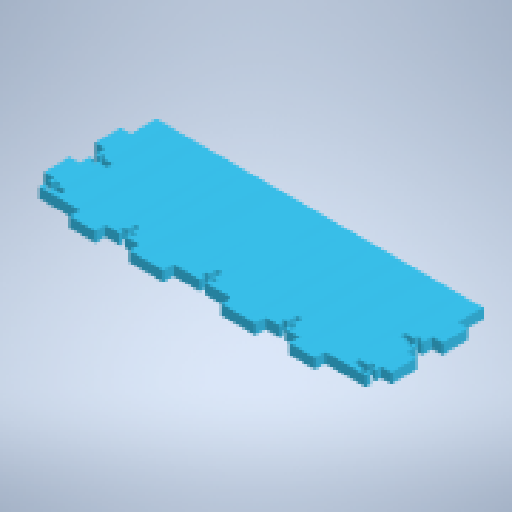
# Autodesk Inventor part: задняя стенка
Saved by Autodesk Inventor 2024.2 (Build 282272000, 272)
## iProperties
Created: 2026-02-22
Part Number: задняя стенка
Material: Типовые
Document SubType Name: Modeling
Designer: Service
Density: 1 g/cm^3
Appearance: Бирюзовый
Author: Service
Autodesk Inventor part; units mm, degrees
ref_plane "YZ Plane" through (0, 0, 0) normal (1, 0, 0) x (0, 1, 0)
ref_plane "XZ Plane" through (0, 0, 0) normal (0, 1, 0) x (-1, 0, 0)
ref_plane "XY Plane" through (0, 0, 0) normal (0, 0, 1) x (1, 0, 0)
sketch "Эскиз1" plane through (0, 0, 0) normal (0, 1, 0) x (-1, 0, 0)
  line L0 (-293.7591, 342.3304) -> (-89.7591, 342.3304)
  line L1 (-89.7591, 342.3304) -> (-89.7591, 402.3304)
  line L2 (-89.7591, 402.3304) -> (-293.7591, 402.3304)
  line L3 (-293.7591, 402.3304) -> (-293.7591, 342.3304)
  line L4 (-293.7591, 387.3304) -> (-287.7591, 387.3304)
  line L5 (-287.7591, 387.3304) -> (-287.7591, 402.3304)
  line L6 (-287.7591, 402.3304) -> (-293.7591, 402.3304)
  line L7 (-293.7591, 402.3304) -> (-293.7591, 387.3304)
  line L8 (-287.7591, 387.3304) -> (-293.7591, 387.3304)
  line L9 (-293.7591, 387.3304) -> (-293.7591, 372.3304)
  line L10 (-293.7591, 372.3304) -> (-287.7591, 372.3304)
  line L11 (-287.7591, 372.3304) -> (-287.7591, 387.3304)
  line L12 (-293.7591, 372.3304) -> (-287.7591, 372.3304)
  line L13 (-287.7591, 372.3304) -> (-287.7591, 357.3304)
  line L14 (-287.7591, 357.3304) -> (-293.7591, 357.3304)
  line L15 (-293.7591, 357.3304) -> (-293.7591, 372.3304)
  line L16 (-287.7591, 357.3304) -> (-293.7591, 357.3304)
  line L17 (-293.7591, 357.3304) -> (-293.7591, 342.3304)
  line L18 (-293.7591, 342.3304) -> (-287.7591, 342.3304)
  line L19 (-287.7591, 342.3304) -> (-287.7591, 357.3304)
  line L20 (-95.7591, 402.3304) -> (-89.7591, 402.3304)
  line L21 (-89.7591, 402.3304) -> (-89.7591, 387.3304)
  line L22 (-89.7591, 387.3304) -> (-95.7591, 387.3304)
  line L23 (-95.7591, 387.3304) -> (-95.7591, 402.3304)
  line L24 (-95.7591, 387.3304) -> (-89.7591, 387.3304)
  line L25 (-89.7591, 387.3304) -> (-89.7591, 372.3304)
  line L26 (-89.7591, 372.3304) -> (-95.7591, 372.3304)
  line L27 (-95.7591, 372.3304) -> (-95.7591, 387.3304)
  line L28 (-95.7591, 372.3304) -> (-89.7591, 372.3304)
  line L29 (-89.7591, 372.3304) -> (-89.7591, 357.3304)
  line L30 (-89.7591, 357.3304) -> (-95.7591, 357.3304)
  line L31 (-95.7591, 357.3304) -> (-95.7591, 372.3304)
  line L32 (-95.7591, 357.3304) -> (-89.7591, 357.3304)
  line L33 (-89.7591, 357.3304) -> (-89.7591, 342.3304)
  line L34 (-89.7591, 342.3304) -> (-95.7591, 342.3304)
  line L35 (-95.7591, 342.3304) -> (-95.7591, 357.3304)
  line L36 (-119.7591, 396.3304) -> (-119.7591, 402.3304)
  line L37 (-89.7591, 390.8181) -> (-89.7591, 394.8304)
  line L38 (-119.7591, 396.3304) -> (-134.7591, 396.3304)
  line L39 (-134.7591, 396.3304) -> (-134.7591, 402.3304)
  line L40 (-134.7591, 402.3304) -> (-119.7591, 402.3304)
  line L41 (-134.7591, 396.3304) -> (-154.7591, 396.3304)
  line L42 (-154.7591, 396.3304) -> (-154.7591, 402.3304)
  line L43 (-154.7591, 402.3304) -> (-134.7591, 402.3304)
  line L44 (-134.7591, 402.3304) -> (-134.7591, 396.3304)
  line L45 (-191.7591, 402.3304) -> (-154.7591, 402.3304)
  line L46 (-154.7591, 402.3304) -> (-154.7591, 396.3304)
  line L47 (-119.7591, 396.3304) -> (-89.7591, 396.3304)
  line L48 (-89.7591, 396.3304) -> (-89.7591, 402.3304)
  line L49 (-89.7591, 402.3304) -> (-119.7591, 402.3304)
  line L50 (-119.7591, 402.3304) -> (-119.7591, 396.3304)
  line L51 (-154.7591, 396.3304) -> (-174.7591, 396.3304)
  line L52 (-174.7591, 396.3304) -> (-174.7591, 402.3304)
  line L53 (-174.7591, 402.3304) -> (-154.7591, 402.3304)
  line L54 (-154.7591, 402.3304) -> (-154.7591, 396.3304)
  line L55 (-293.7591, 394.4817) -> (-263.7591, 394.4817)
  line L56 (-263.7591, 394.4817) -> (-263.7591, 402.3304)
  line L57 (-263.7591, 402.3304) -> (-293.7591, 402.3304)
  line L58 (-293.7591, 402.3304) -> (-293.7591, 394.4817)
  line L59 (-263.7591, 394.4817) -> (-248.7591, 394.4817)
  line L60 (-248.7591, 394.4817) -> (-248.7591, 402.3304)
  line L61 (-248.7591, 402.3304) -> (-263.7591, 402.3304)
  line L62 (-263.7591, 402.3304) -> (-263.7591, 394.4817)
  line L63 (-248.7591, 394.4817) -> (-228.7591, 394.4817)
  line L64 (-228.7591, 394.4817) -> (-228.7591, 402.3304)
  line L65 (-228.7591, 402.3304) -> (-248.7591, 402.3304)
  line L66 (-248.7591, 402.3304) -> (-248.7591, 394.4817)
  line L67 (-228.7591, 394.4817) -> (-208.7591, 394.4817)
  line L68 (-208.7591, 394.4817) -> (-208.7591, 402.3304)
  line L69 (-208.7591, 402.3304) -> (-228.7591, 402.3304)
  line L70 (-228.7591, 402.3304) -> (-228.7591, 394.4817)
  line L71 (-174.7591, 396.3304) -> (-210.3193, 394.4817)
  line L72 (-263.7591, 402.3304) -> (-248.7591, 402.3304)
  line L73 (-248.7591, 402.3304) -> (-248.7591, 417.3304)
  line L74 (-248.7591, 417.3304) -> (-263.7591, 417.3304)
  line L75 (-263.7591, 417.3304) -> (-263.7591, 402.3304)
  line L76 (-228.7591, 402.3304) -> (-208.7591, 402.3304)
  line L77 (-208.7591, 402.3304) -> (-208.7591, 417.3304)
  line L78 (-208.7591, 417.3304) -> (-228.7591, 417.3304)
  line L79 (-228.7591, 417.3304) -> (-228.7591, 402.3304)
  line L80 (-174.7591, 402.3304) -> (-154.7591, 402.3304)
  line L81 (-154.7591, 402.3304) -> (-154.7591, 417.3304)
  line L82 (-154.7591, 417.3304) -> (-174.7591, 417.3304)
  line L83 (-174.7591, 417.3304) -> (-174.7591, 402.3304)
  line L84 (-134.7591, 402.3304) -> (-119.7591, 402.3304)
  line L85 (-119.7591, 402.3304) -> (-119.7591, 417.3304)
  line L86 (-119.7591, 417.3304) -> (-134.7591, 417.3304)
  line L87 (-134.7591, 417.3304) -> (-134.7591, 402.3304)
  line L88 (-95.7591, 402.3304) -> (-95.7591, 411.3304)
  line L89 (-95.7591, 411.3304) -> (-95.7591, 402.3304)
  line L90 (-95.7591, 411.3304) -> (-287.7591, 411.3304)
  line L91 (-287.7591, 411.3304) -> (-287.7591, 402.3304)
  line L92 (-240.2591, 411.3304) -> (-237.2591, 411.3304)
  line L93 (-237.2591, 411.3304) -> (-237.2591, 401.3304)
  line L94 (-237.2591, 401.3304) -> (-240.2591, 401.3304)
  line L95 (-240.2591, 401.3304) -> (-240.2591, 411.3304)
  line L96 (-235.2591, 409.3304) -> (-242.2591, 409.3304)
  line L97 (-242.2591, 409.3304) -> (-242.2591, 406.9304)
  line L98 (-242.2591, 406.9304) -> (-235.2591, 406.9304)
  line L99 (-235.2591, 406.9304) -> (-235.2591, 409.3304)
  line L100 (-190.2591, 411.3304) -> (-190.2591, 401.3304)
  line L101 (-190.2591, 401.3304) -> (-193.2591, 401.3304)
  line L102 (-193.2591, 401.3304) -> (-193.2591, 411.3304)
  line L103 (-188.2591, 408.4317) -> (-195.2591, 408.4317)
  line L104 (-195.2591, 408.4317) -> (-195.2591, 406.0317)
  line L105 (-195.2591, 406.0317) -> (-188.2591, 406.0317)
  line L106 (-188.2591, 406.0317) -> (-188.2591, 408.4317)
  line L107 (-143.2591, 411.3304) -> (-143.2591, 401.3304)
  line L108 (-143.2591, 401.3304) -> (-146.2591, 401.3304)
  line L109 (-146.2591, 401.3304) -> (-146.2591, 404.4797)
  line L110 (-141.2591, 409.3304) -> (-148.2591, 409.3304)
  line L111 (-148.2591, 409.3304) -> (-148.2591, 406.9304)
  line L112 (-148.2591, 406.9304) -> (-141.2591, 406.9304)
  line L113 (-141.2591, 406.9304) -> (-141.2591, 409.3304)
  line L114 (-146.2591, 401.3304) -> (-146.2591, 411.3304)
  point P0 (0, 0)
  point P1 (-290.7591, 402.3304)
  point P2 (-290.7591, 387.3304)
  point P3 (-340.6033, 461.9261)
  point P4 (-287.7591, 394.4817)
  point P5 (-89.7591, 396.3304)
  point P6 (-95.7591, 396.3304)
  point P7 (-208.7591, 402.3304)
  point P8 (-228.7591, 402.3304)
  point P9 (-248.7591, 402.3304)
  point P10 (-208.7591, 402.3304)
  point P11 (-208.7591, 394.5628)
  point P12 (-119.7591, 411.3304)
  point P13 (-134.7591, 411.3304)
  point P14 (-154.7591, 411.3304)
  point P15 (-174.7591, 411.3304)
  point P16 (-208.7591, 411.3304)
  point P17 (-228.7591, 411.3304)
  point P18 (-248.7591, 411.3304)
  point P19 (-263.7591, 411.3304)
  point P20 (-240.2591, 406.3304)
  point P21 (-238.7591, 406.9304)
  point P22 (-238.7591, 409.3304)
  point P23 (-278.7591, 402.3304)
  point P24 (-237.2591, 409.3304)
  point P25 (-237.2591, 406.9304)
  point P26 (-240.2591, 406.9304)
  point P27 (-240.2591, 409.3304)
  point P28 (-248.7591, 409.8304)
  point P29 (-193.2591, 406.3304)
  point P30 (-191.7591, 406.0317)
  point P31 (-191.7591, 408.4317)
  point P32 (-146.2591, 402.905)
  point P33 (-144.7591, 406.9304)
  point P34 (-144.7591, 409.3304)
  point P35 (-190.2591, 408.4317)
  point P36 (-190.2591, 406.0317)
  point P37 (-193.2591, 406.0317)
  point P38 (-193.2591, 408.4317)
  point P39 (-146.2591, 406.9304)
  point P40 (-146.2591, 409.3304)
  point P41 (-143.2591, 409.3304)
  point P42 (-143.2591, 406.9304)
  dimension "d0" = 204
  dimension "d1" = 60
  dimension "d2" = 6
  dimension "d3" = 15
  dimension "d4" = 15
  dimension "d5" = 6
  dimension "d6" = 6
  dimension "d8" = 15
  dimension "d9" = 20
  dimension "d11" = 30
  dimension "d12" = 20
  dimension "d23" = 20
  dimension "d24" = 20
  dimension "d25" = 15
  dimension "d26" = 30
  dimension "d29" = 15
  dimension "d30" = 15
  dimension "d31" = 15
  dimension "d32" = 15
  dimension "d33" = 7
  dimension "d34" = 3
  dimension "d35" = 2
  dimension "d36" = 2.4
  dimension "d37" = 10
  dimension "d38" = 9
  dimension "d39" = 8.5
  dimension "d40" = 7
  dimension "d41" = 3
  dimension "d42" = 2
  dimension "d43" = 2.4
  dimension "d44" = 10
  dimension "d45" = 7
  dimension "d46" = 3
  dimension "d47" = 2
  dimension "d48" = 2.4
  dimension "d49" = 10
  dimension "d50" = 2
  dimension "d51" = 2
  dimension "d52" = 15.5
  dimension "d53" = 15
  dimension "d54" = 20
  dimension "d55" = 20
  dimension "d56" = 15
  dimension "d57" = 28.5
  constraints: 228 end point, 51 parallel, 30 perpendicular, 28 horizontal, 16 midpoint, 14 point on line, 5 collinear, 2 vertical, 11 other
  measures "d0" distance between parallel lines of L1 L3
  measures "d2" distance between parallel lines of L17 L19
  measures "d3" distance of point (-290.759, 402.33) point (-290.759, 387.33)
  measures "d4" distance of L22.end L20.start
  measures "d5" distance between parallel lines of L23 L1
  measures "d6" distance between parallel lines of L40 L38
  measures "d8" distance of L36.start L38.end
  measures "d9" distance of L38.end L41.end
  measures "d11" distance of L36.start L47.end
  measures "d12" distance of L41.end L51.end
  measures "d23" distance of L67.start L67.end
  measures "d24" distance of L59.end L63.end
  measures "d25" distance of L55.end L59.end
  measures "d26" distance of L55.start L55.end
  measures "d29" distance of L84.end L85.end
  measures "d30" distance of L80.end L81.end
  measures "d31" distance of L76.end L77.end
  measures "d32" distance of L72.end L73.end
  measures "d33" distance of L96.start L96.end
  measures "d34" distance between parallel lines of L95 L93
  measures "d35" distance from line of point (-240.259, 406.33) L97
  measures "d36" distance of point (-238.759, 406.93) point (-238.759, 409.33)
  measures "d37" distance of L92.end L93.end
  measures "d38" distance from line of L90 point (-278.759, 402.33)
  measures "d39" distance from line of point (-248.759, 409.83) L95
  measures "d40" distance of L103.start L103.end
  measures "d41" distance between parallel lines of L102 L100
  measures "d42" distance from line of point (-193.259, 406.33) L104
  measures "d43" distance of point (-191.759, 406.032) point (-191.759, 408.432)
  measures "d44" distance of L100.start L100.end
  measures "d45" distance of L110.start L110.end
  measures "d46" distance between parallel lines of L109 L107
  measures "d47" distance from line of point (-146.259, 402.905) L111
  measures "d48" distance of point (-144.759, 406.93) point (-144.759, 409.33)
  measures "d49" distance of L107.start L107.end
  measures "d50" distance between parallel lines of L90 L96
  measures "d51" distance between parallel lines of L90 L110
  measures "d52" distance between parallel lines of L77 L102
  measures "d53" distance of L73.end L74.end
  measures "d54" distance of L77.end L78.end
  measures "d55" distance of L81.end L82.end
  measures "d56" distance of L85.end L86.end
  measures "d57" distance between parallel lines of L83 L114
extrude "Выдавливание1" add sketch "Эскиз1" along normal blind 6 contours L19 L13 L11 L5 L55 L59 L63 L67 L68 L71 L51 L41 L38 L47 L23 L27 L31 L35 L0 | L3 L10 L13 L14 | L31 L26 L1 L30 | L3 L55 L5 L4 | L3 L2 L5 L55 | L23 L47 L1 L22 | L5 L2 L56 L55 | L47 L36 L2 L23 | L23 L2 L1 L47 | L91 L90 L75 L2 | L56 L2 L60 L59 | L2 L85 L90 L88 | L38 L39 L2 L36 | L75 L90 L73 L2 | L60 L2 L95 L94 L93 L64 L63 | L2 L87 L90 L85 | L41 L42 L2 L109 L108 L107 L39 | L73 L90 L95 L96 L97 L98 L2 | L75 L74 L73 L90 | L64 L2 L68 L71 L67 | L2 L107 L112 L113 L110 L90 L87 | L90 L87 L86 L85 | L51 L52 L2 L42 | L79 L90 L77 L2 | L2 L93 L98 L99 L96 L90 L79 | L71 L68 L67 | L107 L108 L109 L2 | L81 L90 L114 L110 L111 L112 L109 L2 | L2 L83 L90 L81 | L71 L68 L2 L102 L101 L100 L52 | L77 L90 L102 L103 L104 L105 L2 | L79 L78 L77 L90 | L2 L100 L105 L106 L103 L90 L83 | L90 L83 L82 L81
sketch "Эскиз2" plane through (0, 0, 0) normal (0, -1, 0) x (1, 0, 0)
  line L0 (287.7591, 378.3304) -> (277.7591, 378.3304)
  line L1 (277.7591, 378.3304) -> (277.7591, 381.3304)
  line L2 (277.7591, 381.3304) -> (287.7591, 381.3304)
  line L3 (287.7591, 381.3304) -> (287.7591, 378.3304)
  line L4 (283.3591, 376.3304) -> (285.7591, 376.3304)
  line L5 (285.7591, 376.3304) -> (285.7591, 383.3304)
  line L6 (285.7591, 383.3304) -> (283.3591, 383.3304)
  line L7 (283.3591, 383.3304) -> (283.3591, 376.3304)
  line L8 (287.7591, 387.3304) -> (287.7591, 372.3304) projected
  line L9 (293.7591, 387.3304) -> (287.7591, 387.3304) projected
  line L10 (290.153, 393.3304) -> (255.2368, 393.3304) construction
  line L11 (287.7591, 342.3304) -> (95.7591, 342.3304) construction
  line L12 (191.7591, 342.3304) -> (191.7591, 378.3304) construction
  line L13 (287.7591, 408.3304) -> (277.7591, 408.3304)
  line L14 (277.7591, 408.3304) -> (277.7591, 405.3304)
  line L15 (277.7591, 405.3304) -> (287.7591, 405.3304)
  line L16 (287.7591, 405.3304) -> (287.7591, 408.3304)
  line L17 (283.3591, 410.3304) -> (285.7591, 410.3304)
  line L18 (285.7591, 410.3304) -> (285.7591, 403.3304)
  line L19 (285.7591, 403.3304) -> (283.3591, 403.3304)
  line L20 (283.3591, 403.3304) -> (283.3591, 410.3304)
  line L21 (287.7591, 399.3304) -> (287.7591, 414.3304)
  line L22 (293.7591, 399.3304) -> (287.7591, 399.3304)
  line L23 (95.7591, 378.3304) -> (105.7591, 378.3304)
  line L24 (105.7591, 378.3304) -> (105.7591, 381.3304)
  line L25 (105.7591, 381.3304) -> (95.7591, 381.3304)
  line L26 (95.7591, 381.3304) -> (95.7591, 378.3304)
  line L27 (100.1591, 376.3304) -> (97.7591, 376.3304)
  line L28 (97.7591, 376.3304) -> (97.7591, 383.3304)
  line L29 (97.7591, 383.3304) -> (100.1591, 383.3304)
  line L30 (100.1591, 383.3304) -> (100.1591, 376.3304)
  line L31 (95.7591, 408.3304) -> (105.7591, 408.3304)
  line L32 (105.7591, 408.3304) -> (105.7591, 405.3304)
  line L33 (105.7591, 405.3304) -> (95.7591, 405.3304)
  line L34 (95.7591, 405.3304) -> (95.7591, 408.3304)
  line L35 (97.7591, 410.3304) -> (97.7591, 403.3304)
  line L36 (97.7591, 403.3304) -> (100.1591, 403.3304)
  line L37 (100.1591, 403.3304) -> (100.1591, 410.3304)
  line L38 (100.1591, 410.3304) -> (97.7591, 410.3304)
  point P0 (0, 0)
  point P1 (95.7591, 387.3304)
  point P2 (95.7591, 399.3304)
  point P3 (283.3591, 381.3304)
  point P4 (283.3591, 378.3304)
  point P5 (285.7591, 378.3304)
  point P6 (285.7591, 381.3304)
  point P7 (283.3591, 408.3304)
  point P8 (283.3591, 405.3304)
  point P9 (285.7591, 405.3304)
  point P10 (285.7591, 408.3304)
  point P11 (97.7591, 408.3304)
  point P12 (97.7591, 405.3304)
  point P13 (100.1591, 405.3304)
  point P14 (100.1591, 408.3304)
  point P15 (100.1591, 378.3304)
  point P16 (100.1591, 381.3304)
  point P17 (97.7591, 381.3304)
  point P18 (97.7591, 378.3304)
  dimension "d58" = 10
  dimension "d59" = 3
  dimension "d60" = 7
  dimension "d61" = 2
  dimension "d62" = 2.4
  dimension "d63" = 2
  dimension "d64" = 6
  dimension "d65" = 12
  constraints: 72 end point, 29 symmetric about line, 4 parallel, 3 horizontal, 2 perpendicular, 1 collinear, 1 midpoint, 1 vertical
  measures "d58" distance of L0.start L0.end
  measures "d59" distance of L0.end L1.end
  measures "d60" distance of L6.end L4.start
  measures "d61" distance between parallel lines of L0 L4
  measures "d62" distance between parallel lines of L5 L7
  measures "d63" distance between parallel lines of L8 L5
  measures "d64" distance between parallel lines of L9 L2
  measures "d65" distance between parallel lines of L2 L10
extrude "Выдавливание2" cut sketch "Эскиз2" against normal blind 6
